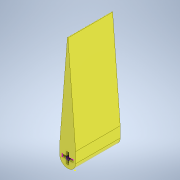
# Autodesk Inventor part: Bistable Flipper 2
Saved by Autodesk Inventor 2020 (Build 240168000, 168)
## iProperties
Created: 2019-11-08
Part Number: Bistable Flipper 2
Material: Stainless Steel, Polished
Document SubType Name: Modeling
Designer: camde
Density: 8 g/cm^3
Appearance: Yellow
Mass: 5335.57 g
Surface Area: 780.011 cm^2
Volume: 666.946 cm^3
Author: camde
Autodesk Inventor part; units mm, degrees
ref_plane "YZ Plane" through (0, 0, 0) normal (1, 0, 0) x (0, 1, 0)
ref_plane "XZ Plane" through (0, 0, 0) normal (0, 1, 0) x (-1, 0, 0)
ref_plane "XY Plane" through (0, 0, 0) normal (0, 0, 1) x (1, 0, 0)
sketch "Sketch1" plane through (0, 0, 0) normal (0, 0, 1) x (1, 0, 0)
  line L0 (-37.1271, 279.7291) -> (1.4084, 279.7291)
  line L1 (1.4084, 279.7291) -> (1.4084, -4.9324)
  line L2 (1.4084, -4.9324) -> (-37.1271, -4.9324)
  line L3 (-37.1271, -4.9324) -> (-37.1271, 279.7291)
  point P0 (0, 0)
  dimension "d0" = 38.5354
  dimension "d1" = 284.6614
  constraints: 8 end point, 2 parallel, 1 horizontal, 1 perpendicular
  measures "d0" distance of L1.end L2.end
  measures "d1" distance of L0.end L1.end
extrude "Extrusion1" add sketch "Sketch1" along normal blind 108.8571
sketch "Sketch2" plane through (0, 0, 108.8571) normal (0, 0, 1) x (1, 0, 0)
  line L0 (-37.1271, -4.9324) -> (1.4084, -4.9324) projected
  line L1 (-17.8594, -4.9324) -> (-17.8594, 16.8391) construction
  circle A0 centre (-17.8594, 16.8391) radius 13.6071 construction
  line L2 (-17.8594, 16.8391) -> (-20.753, 30.135) construction
  line L3 (-17.8594, 16.8391) -> (-14.9657, 30.135) construction
  line L4 (-20.753, 30.135) -> (-14.9657, 30.135)
  line L5 (-17.8594, 16.8391) -> (-31.1553, 13.9454) construction
  line L6 (-31.1553, 13.9454) -> (-31.1553, 19.7327)
  line L7 (-17.8594, 16.8391) -> (-14.9657, 3.5432) construction
  line L8 (-14.9657, 3.5432) -> (-20.753, 3.5432)
  line L9 (-17.8594, 16.8391) -> (-4.5634, 19.7327) construction
  line L10 (-4.5634, 19.7327) -> (-4.5634, 13.9454)
  line L11 (-20.753, 30.135) -> (-20.753, 19.7327)
  line L12 (-20.753, 13.9454) -> (-20.753, 3.5432)
  line L13 (-31.1553, 13.9454) -> (-20.753, 13.9454)
  line L14 (-14.9657, 13.9454) -> (-4.5634, 13.9454)
  line L15 (-14.9657, 3.5432) -> (-14.9657, 13.9454)
  line L16 (-14.9657, 19.7327) -> (-14.9657, 30.135)
  line L17 (-14.9657, 19.7327) -> (-4.5634, 19.7327)
  line L18 (-31.1553, 19.7327) -> (-20.753, 19.7327)
  point P0 (0, 0)
  dimension "d4" = 21.7714
  dimension "d5" = 27.2143
  dimension "d18" = 360
  constraints: 36 end point, 4 parallel, 3 horizontal, 3 vertical, 2 perpendicular, 2 point on circle, 1 centre point, 1 coincident, 1 midpoint, 21 other
  measures "d4" distance of L1.start L1.end
  measures "d5" diameter of A0
fillet "Fillet1" radius 19.2677 2 edges at (1.4084, -4.9324, 54.4286) (-37.1271, -4.9324, 54.4286)
chamfer "Chamfer1" distance 19.2677 distance2 239.4857 1 edges at (-37.1271, 279.7291, 54.4286) measured on face at (-11.4368, 279.7291, 36.2857)
chamfer "Chamfer2" distance 239.4857 distance2 19.2677 1 edges at (1.4084, 279.7291, 54.4286) measured on face at (1.4084, 102.7999, 36.2857)
sketch "Sketch3" plane through (0, 0, 108.8571) normal (0, 0, 1) x (1, 0, 0)
  point P0 (0, 0)
extrude "Extrusion3" cut sketch "Sketch2" against normal blind 25.4
sketch "Sketch4" plane through (0, 0, 108.8571) normal (0, 0, 1) x (1, 0, 0)
  line L0 (-31.1553, 19.7327) -> (-31.1553, 13.9454) projected
  line L1 (-31.1553, 13.9454) -> (-31.1553, 19.7327) projected
  line L2 (-31.1553, 16.8391) -> (-13.0927, 16.8391) construction
  line L3 (-4.5634, 19.7327) -> (-14.9657, 19.7327) projected
  circle A0 centre (-17.8594, 16.8391) radius 4.0922
  point P0 (0, 0)
  constraints: 2 end point, 1 horizontal, 1 midpoint, 1 point on line, 3 other
fillet "Fillet3" radius 0.6802 2 edges at (-17.8593, 279.7291, 54.4286) (-17.8594, 279.7291, 54.4286)
body "Solid1"
